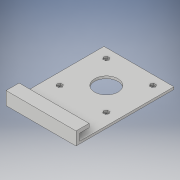
# Autodesk Inventor part: Stand
Saved by Autodesk Inventor 2018 (Build 220112000, 112)
## iProperties
Created: 2017-04-07
Part Number: Stand
Material: Generic
Document SubType Name: Modeling
Designer: klyu
Density: 1 g/cm^3
Appearance: Default
Author: klyu
Autodesk Inventor part; units mm, degrees
ref_plane "YZ Plane" through (0, 0, 0) normal (1, 0, 0) x (0, 1, 0)
ref_plane "XZ Plane" through (0, 0, 0) normal (0, 1, 0) x (-1, 0, 0)
ref_plane "XY Plane" through (0, 0, 0) normal (0, 0, 1) x (1, 0, 0)
sketch "Sketch1" plane through (0, 0, 0) normal (0, 1, 0) x (-1, 0, 0)
  line L0 (0, 0) -> (150, 0)
  line L1 (150, 0) -> (150, -210)
  line L2 (150, -210) -> (0, -210)
  line L3 (0, -210) -> (0, 0)
  dimension "d11" = 150
  dimension "d12" = 210
  constraints: 8 end point, 2 parallel, 1 horizontal, 1 perpendicular
  measures "d11" distance between parallel lines of L3 L1
  measures "d12" distance between parallel lines of L2 L0
extrude "Extrusion1" add sketch "Sketch1" along normal blind 5
sketch "Sketch2" plane through (0, 5, 0) normal (0, 1, 0) x (1, 0, 0)
  line L0 (-150, 0) -> (0, 0) projected
  line L1 (-150, 210) -> (-150, 0) projected
  line L2 (0, 0) -> (-150, 0)
  line L3 (-150, 0) -> (-150, 8)
  line L4 (-150, 8) -> (0, 8)
  line L5 (0, 8) -> (0, 0)
  dimension "d13" = 8
  constraints: 8 end point, 2 parallel, 1 horizontal, 1 perpendicular, 1 point on line
  measures "d13" distance between parallel lines of L0 L4
extrude "Extrusion2" add sketch "Sketch2" along normal blind 23
sketch "Sketch3" plane through (0, 5, -8) normal (0, 0, -1) x (-1, 0, 0)
  line L0 (150, 23) -> (0, 23) projected
  line L1 (150, -5) -> (150, 23) projected
  line L2 (0, 23) -> (150, 23)
  line L3 (150, 23) -> (150, 15)
  line L4 (150, 15) -> (0, 15)
  line L5 (0, 15) -> (0, 23)
  point P0 (0, -5)
  dimension "d14" = 8
  constraints: 8 end point, 2 parallel, 1 horizontal, 1 perpendicular, 1 point on line
  measures "d14" distance between parallel lines of L4 L0
extrude "Extrusion3" add sketch "Sketch3" along normal blind 20
sketch "Sketch6" plane through (0, 5, 0) normal (0, 1, 0) x (1, 0, 0)
  line L0 (-150, 8) -> (0, 8) projected
  line L1 (-75, 8) -> (-75, 210)
  line L2 (0, 210) -> (-150, 210) projected
  line L3 (-150, 210) -> (-150, 8) projected
  line L4 (-150, 140) -> (0, 140)
  line L5 (0, 8) -> (0, 210) projected
  circle A0 centre (-125, 90) radius 3.2
  circle A1 centre (-125, 190) radius 3.2
  circle A2 centre (-25, 190) radius 3.2
  circle A3 centre (-25, 90) radius 3.2
  line L6 (-150, 0) -> (0, 0) projected
  dimension "d44" = 50
  dimension "d45" = 6.4
  dimension "d46" = 50
  dimension "d64" = 140
  constraints: 4 centre point, 4 end point, 3 midpoint, 3 point on line, 1 horizontal, 1 vertical, 3 other
  measures "d44" distance from line of L1 A1.centre
  measures "d45" diameter of A1
  measures "d46" distance from line of L4 A1.centre
  measures "d64" distance between parallel lines of L6 L4
hole "Hole2" at (-25, 5, -190) at (-25, 5, -90) at (-125, 5, -90) at (-125, 5, -190) direction (0, -1, 0) diameter 6.4 end through all counterbore diameter 9 counterbore depth 3.8
sketch "Sketch5" plane through (0, 5, 0) normal (0, 1, 0) x (1, 0, 0)
  line L0 (-27.8868, 195) -> (-22.1132, 195)
  line L1 (-22.1132, 195) -> (-19.2265, 190)
  line L2 (-19.2265, 190) -> (-22.1132, 185)
  line L3 (-22.1132, 185) -> (-27.8868, 185)
  line L4 (-27.8868, 185) -> (-30.7735, 190)
  line L5 (-30.7735, 190) -> (-27.8868, 195)
  line L6 (-27.8868, 85) -> (-30.7735, 90)
  line L7 (-30.7735, 90) -> (-27.8868, 95)
  line L8 (-27.8868, 95) -> (-22.1132, 95)
  line L9 (-22.1132, 95) -> (-19.2265, 90)
  line L10 (-19.2265, 90) -> (-22.1132, 85)
  line L11 (-22.1132, 85) -> (-27.8868, 85)
  line L12 (-127.8868, 185) -> (-130.7735, 190)
  line L13 (-130.7735, 190) -> (-127.8868, 195)
  line L14 (-127.8868, 195) -> (-122.1132, 195)
  line L15 (-122.1132, 195) -> (-119.2265, 190)
  line L16 (-119.2265, 190) -> (-122.1132, 185)
  line L17 (-122.1132, 185) -> (-127.8868, 185)
  line L18 (-150, 210) -> (0, 210) projected
  line L19 (-75, 210) -> (-75, 30.6019)
  line L20 (-127.8868, 85) -> (-130.7735, 90)
  line L21 (-130.7735, 90) -> (-127.8868, 95)
  line L22 (-127.8868, 95) -> (-122.1132, 95)
  line L23 (-122.1132, 95) -> (-119.2265, 90)
  line L24 (-119.2265, 90) -> (-122.1132, 85)
  line L25 (-122.1132, 85) -> (-127.8868, 85)
  line L26 (-150, 210) -> (-150, 8) projected
  line L27 (-146.8054, 140) -> (0, 140)
  line L28 (0, 210) -> (0, 0) projected
  line L29 (-150, 0) -> (0, 0) projected
  point P0 (-25, 190)
  point P1 (-25, 90)
  point P2 (-125, 190)
  point P3 (-125, 90)
  dimension "d34" = 10
  dimension "d54" = 10
  dimension "d55" = 10
  dimension "d56" = 10
  dimension "d57" = 100
  dimension "d58" = 100
  dimension "d65" = 140
  constraints: 52 end point, 5 horizontal, 4 symmetric about line, 1 midpoint, 1 point on line, 1 vertical, 52 other
  measures "d34" distance between parallel lines of L1 L4
  measures "d54" distance between parallel lines of L16 L13
  measures "d55" distance between parallel lines of L21 L24
  measures "d56" distance between parallel lines of L10 L7
  measures "d57" distance of point (-125, 90) point (-125, 190)
  measures "d58" distance of point (-25, 190) point (-125, 190)
  measures "d65" distance between parallel lines of L29 L27
extrude "Extrusion6" cut sketch "Sketch5" against normal blind 3.8 contours L0 L1 L2 L3 L4 L5 | L6 L7 L8 L9 L10 L11 | L12 L13 L14 L15 L16 L17 | L20 L21 L22 L23 L24 L25
sketch "Sketch7" plane through (0, 5, 0) normal (0, 1, 0) x (1, 0, 0)
  circle A0 centre (-75, 140) radius 27.9443
  line L0 (-150, 140) -> (0, 140)
  line L1 (-150, 210) -> (0, 210) projected
  line L2 (-75, 210) -> (-75, 0)
  line L3 (0, 210) -> (0, 0) projected
  line L4 (-150, 210) -> (0, 210)
  line L5 (0, 210) -> (0, 0)
  line L6 (0, 0) -> (-150, 0)
  line L7 (-150, 0) -> (-150, 210)
  line L8 (0, 8) -> (0, 210) projected
  line L9 (-150, 210) -> (-150, 8) projected
  line L10 (0, 210) -> (-150, 210) projected
  line L11 (-150, 0) -> (0, 0) projected
  dimension "d66" = 140
  constraints: 12 end point, 5 midpoint, 3 parallel, 3 point on line, 2 horizontal, 1 centre point, 1 coincident, 1 perpendicular, 1 vertical
  measures "d66" distance between parallel lines of L6 L0
hole "Hole3" at (-75, 5, -140) direction (0, -1, 0) diameter 50 end through all
body "Solid1"
